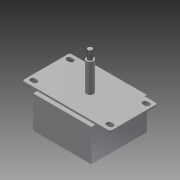
# Autodesk Inventor part: JLF-TP-8YT_body
Saved by Autodesk Inventor 2013 (Build 170138000, 138)
## iProperties
Created: 2013-01-27
Part Number: JLF-TP-8YT_body
Material: Steel AISI 4620
Document SubType Name: Modeling
Designer: xylzlyx
Density: 1 g/cm^3
Author: xylzlyx
Autodesk Inventor part; units mm, degrees
ref_plane "YZ Plane" through (0, 0, 0) normal (1, 0, 0) x (0, 1, 0)
ref_plane "XZ Plane" through (0, 0, 0) normal (0, 1, 0) x (-1, 0, 0)
ref_plane "XY Plane" through (0, 0, 0) normal (0, 0, 1) x (1, 0, 0)
sketch "JoystickMount" plane through (0, 0, 0) normal (0, 0, 1) x (1, 0, 0)
  line L0 (-49, 26.5) -> (49, 26.5)
  line L1 (49, 26.5) -> (49, -26.5)
  line L2 (49, -26.5) -> (-49, -26.5)
  line L3 (-49, -26.5) -> (-49, 26.5)
  point P0 (0, 0)
  point P1 (-49, 0)
  point P2 (0, 26.5)
  point P3 (0, -26.5)
  point P4 (49, 0)
  dimension "d0" = 53
  dimension "d2" = 98
  constraints: 8 end point, 4 midpoint, 2 horizontal alignment, 2 parallel, 2 vertical alignment, 1 horizontal, 1 perpendicular
  measures "d0" distance of L2.end L0.start
  measures "d2" distance of L0.start L0.end
extrude "JoystickMountPlate" add sketch "JoystickMount" against normal blind 2
fillet "MountPlateCornerFillet" radius 2 4 edges at (49, 26.5, -1) (-49, 26.5, -1) (-49, -26.5, -1) (49, -26.5, -1)
sketch "BodySketch" plane through (0, 0, -2) normal (0, 0, -1) x (-1, 0, 0)
  line L0 (-32.5, 31) -> (32.5, 31)
  line L1 (32.5, 31) -> (32.5, -31)
  line L2 (32.5, -31) -> (-32.5, -31)
  line L3 (-32.5, -31) -> (-32.5, 31)
  point P0 (0, 0)
  point P1 (-32.5, 0)
  point P2 (0, 31)
  dimension "d6" = 65
  dimension "d8" = 62
  constraints: 8 end point, 2 midpoint, 2 parallel, 1 horizontal, 1 horizontal alignment, 1 perpendicular, 1 vertical alignment
  measures "d6" distance of L0.start L0.end
  measures "d8" distance of L2.end L0.start
extrude "JoystickBody" add sketch "BodySketch" along normal blind 36
sketch "JoystickPostCenter" plane through (0, 0, 0) normal (0, 0, 1) x (1, 0, 0)
  circle A0 centre (0, 0) radius 4
  dimension "d11" = 8
  constraints: 3 coincident, 1 centre point
  measures "d11" diameter of A0
extrude "Shaft" add sketch "JoystickPostCenter" along normal blind 32
sketch "ThreadSketch" plane through (0, 0, 32) normal (0, 0, 1) x (1, 0, 0)
  circle A0 centre (0, 0) radius 4 projected
  circle A1 centre (0, 0) radius 2.5
  dimension "d14" = 5
  constraints: 1 centre point, 1 coincident
  measures "d14" diameter of A1
extrude "ShaftScrew" add sketch "ThreadSketch" along normal blind 10 contours A1
thread "ShaftThread" size "M5x0.8" class "6g" standard "ANSI Metric M Profile" full length
sketch "ObroundMountSketch" plane through (0, 0, 0) normal (0, 0, 1) x (1, 0, 0)
  circle A0 centre (0, 0) radius 4 projected
  arc A1 (-41.25, 17.5) -> (-41.25, 23) centre (-41.25, 20.25) ccw
  arc A2 (-43.75, 23) -> (-43.75, 17.5) centre (-43.75, 20.25) ccw
  line L0 (-43.75, 23) -> (-41.25, 23)
  line L1 (-41.25, 17.5) -> (-43.75, 17.5)
  arc A3 (-41.25, -23) -> (-41.25, -17.5) centre (-41.25, -20.25) ccw
  arc A4 (-43.75, -17.5) -> (-43.75, -23) centre (-43.75, -20.25) ccw
  line L2 (-43.75, -17.5) -> (-41.25, -17.5)
  line L3 (-41.25, -23) -> (-43.75, -23)
  arc A5 (43.75, -23) -> (43.75, -17.5) centre (43.75, -20.25) ccw
  arc A6 (41.25, -17.5) -> (41.25, -23) centre (41.25, -20.25) ccw
  line L4 (41.25, -17.5) -> (43.75, -17.5)
  line L5 (43.75, -23) -> (41.25, -23)
  arc A7 (43.75, 17.5) -> (43.75, 23) centre (43.75, 20.25) ccw
  arc A8 (41.25, 23) -> (41.25, 17.5) centre (41.25, 20.25) ccw
  line L6 (41.25, 23) -> (43.75, 23)
  line L7 (43.75, 17.5) -> (41.25, 17.5)
  line L8 (-42.5, 20.25) -> (-42.5, -20.25) construction
  line L9 (-42.5, -20.25) -> (42.5, -20.25) construction
  point P0 (-42.5, 23)
  point P1 (-42.5, -17.5)
  point P2 (42.5, -17.5)
  point P3 (42.5, 20.25)
  point P4 (42.5, 23)
  point P5 (-42.5, 0)
  point P6 (0, -20.25)
  dimension "d24" = 2.5
  dimension "d25" = 5.5
  dimension "d26" = 5.5
  dimension "d27" = 2.5
  dimension "d28" = 2.5
  dimension "d29" = 5.5
  dimension "d30" = 5.5
  dimension "d31" = 2.5
  dimension "d32" = 2.5
  dimension "d33" = 5.5
  dimension "d34" = 5.5
  dimension "d35" = 2.5
  dimension "d36" = 2.5
  dimension "d37" = 5.5
  dimension "d38" = 5.5
  dimension "d39" = 2.5
  dimension "d40" = 40.5
  dimension "d41" = 85
  constraints: 20 end point, 16 point on circle, 12 tangent, 11 horizontal alignment, 8 centre point, 8 coincident, 7 vertical alignment, 6 midpoint, 1 perpendicular
  measures "d24" distance of point (-41.25, 20.25) point (-43.75, 20.25)
  measures "d25" diameter of A1
  measures "d26" diameter of A2
  measures "d27" distance of L1.start L1.end
  measures "d28" distance of point (-41.25, -20.25) point (-43.75, -20.25)
  measures "d29" diameter of A3
  measures "d30" diameter of A4
  measures "d31" distance of L3.start L3.end
  measures "d32" distance of point (43.75, -20.25) point (41.25, -20.25)
  measures "d33" diameter of A5
  measures "d34" diameter of A6
  measures "d35" distance of L5.start L5.end
  measures "d36" distance of point (43.75, 20.25) point (41.25, 20.25)
  measures "d37" diameter of A7
  measures "d38" diameter of A8
  measures "d39" distance of L7.start L7.end
  measures "d40" distance of L8.start L8.end
  measures "d41" distance of L8.end L9.end
extrude "MountHoles" cut sketch "ObroundMountSketch" against normal blind 2 contours L1 A2 L0 A1 | L3 A4 L2 A3 | L5 A6 L4 A5 | L7 A8 L6 A7
body "Solid1"
